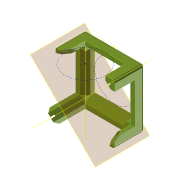
# Autodesk Inventor part: 10_Cube_1x1_v2
Saved by Autodesk Inventor 2019 (Build 230136000, 136)
## iProperties
Created: 2019-07-01
Part Number: 10_Cube_1x1_v2
Material: Generic
Document SubType Name: Modeling
Designer: diederichbenedict
Density: 1 g/cm^3
Appearance: IPHT_Grün
Author: diederichbenedict
Autodesk Inventor part; units mm, degrees
ref_plane "YZ Plane" through (0, 0, 0) normal (1, 0, 0) x (0, 1, 0)
ref_plane "XZ Plane" through (0, 0, 0) normal (0, 1, 0) x (-1, 0, 0)
sketch "Sketch1" plane through (0, 0, 0) normal (0, 0, 1) x (1, 0, 0)
  line L0 (-24.9, 24.9) -> (24.9, 24.9)
  line L1 (24.9, 24.9) -> (24.9, -24.9)
  line L2 (24.9, -24.9) -> (-24.9, -24.9)
  line L3 (-24.9, -24.9) -> (-24.9, 24.9)
  line L4 (-24.9, 24.9) -> (24.9, -24.9) construction
  line L5 (24.9, 24.9) -> (-24.9, -24.9) construction
  line L6 (16.9, 16.9) -> (-16.9, 16.9)
  line L7 (-16.9, 16.9) -> (-16.9, -16.9)
  line L8 (-16.9, -16.9) -> (16.9, -16.9)
  line L9 (16.9, -16.9) -> (16.9, 16.9)
  point P0 (0, 0)
  dimension "d0" = 49.8
  dimension "d1" = 49.8
  dimension "d2" = 8
  constraints: 20 end point, 4 parallel, 2 midpoint, 2 perpendicular, 1 horizontal, 3 other
  measures "d0" distance of L1.end L2.end
  measures "d1" distance of L0.end L1.end
  measures "d2" distance between parallel lines of L0 L6
extrude "Extrusion1" add sketch "Sketch1" along normal blind 8
sketch "Sketch2" plane through (0, 0, 8) normal (0, 0, 1) x (1, 0, 0)
  line L0 (16.9, 16.9) -> (16.9, -16.9) projected
  line L1 (16.9, -16.9) -> (-16.9, -16.9) projected
  line L2 (-16.9, -16.9) -> (-16.9, 16.9) projected
  line L3 (-16.9, 16.9) -> (16.9, 16.9) projected
  line L4 (24.9, 24.9) -> (-24.9, 24.9) projected
  line L5 (-24.9, 24.9) -> (-24.9, -24.9) projected
  line L6 (-24.9, -24.9) -> (24.9, -24.9) projected
  line L7 (24.9, -24.9) -> (24.9, 24.9) projected
  line L8 (16.9, -16.9) -> (24.9, -16.9)
  line L9 (24.9, -16.9) -> (24.9, -24.9)
  line L10 (24.9, -24.9) -> (16.9, -24.9)
  line L11 (16.9, -24.9) -> (16.9, -16.9)
  line L12 (16.9, 16.9) -> (-16.9, 16.9) projected
  line L13 (24.9, 24.9) -> (16.9, 24.9)
  line L14 (16.9, 24.9) -> (16.9, 16.9)
  line L15 (16.9, 16.9) -> (24.9, 16.9)
  line L16 (24.9, 16.9) -> (24.9, 24.9)
  line L17 (-24.9, -24.9) -> (-16.9, -24.9)
  line L18 (-16.9, -24.9) -> (-16.9, -16.9)
  line L19 (-16.9, -16.9) -> (-24.9, -16.9)
  line L20 (-24.9, -16.9) -> (-24.9, -24.9)
  line L21 (-24.9, 24.9) -> (-16.9, 24.9)
  line L22 (-16.9, 24.9) -> (-16.9, 16.9)
  line L23 (-16.9, 16.9) -> (-24.9, 16.9)
  line L24 (-24.9, 16.9) -> (-24.9, 24.9)
  point P0 (0, 0)
  constraints: 32 end point, 8 parallel, 4 horizontal, 4 perpendicular
extrude "Extrusion2" add sketch "Sketch2" along normal blind 16.9 contours L14 L4 L7 L15 | L8 L7 L6 L11 | L23 L5 L4 L22 | L18 L6 L5 L19
sketch "Sketch3" plane through (0, 0, 0) normal (0, 0, -1) x (-1, 0, 0)
  line L0 (24.9, -24.9) -> (24.9, 24.9) construction
  line L1 (24.9, 24.9) -> (-24.9, 24.9) construction
  line L2 (-24.9, -24.9) -> (24.9, -24.9) construction
  line L3 (-24.9, 24.9) -> (-24.9, -24.9) construction
  point P0 (20, 20)
  point P1 (20, -20)
  point P2 (-20, -20)
  point P3 (-20, 20)
  dimension "d_1" = 4.9
  dimension "d96" = 4.9
  dimension "d97" = 4.9
  dimension "d98" = 4.9
  dimension "d99" = 4.9
  dimension "d100" = 4.9
  dimension "d101" = 4.9
  dimension "d102" = 4.9
  measures "d_1" distance from line of L1 point (20, 20)
  measures "d96" distance from line of point (20, 20) L0
  measures "d97" distance from line of point (20, -20) L0
  measures "d98" distance from line of point (20, -20) L2
  measures "d99" distance from line of point (-20, -20) L2
  measures "d100" distance from line of point (-20, -20) L3
  measures "d101" distance from line of point (-20, 20) L3
  measures "d102" distance from line of point (-20, 20) L1
hole "Hole1" at (-20, 20, 0) at (-20, -20, 0) at (20, -20, 0) at (20, 20, 0) direction (0, 0, 1) diameter 2.8 depth 30 tip angle 118 counterbore diameter 5.5 counterbore depth 3.1
sketch "Sketch4" plane through (-24.9, 24.9, 0) normal (0, 1, 0) x (1, 0, 0)
  line L0 (0, 0) -> (49.8, 0) construction
  line L1 (0, 0) -> (0, -24.9) construction
  line L2 (8, -24.9) -> (0, -24.9) construction
  line L3 (8, -8) -> (8, -24.9) construction
  line L4 (41.8, -8) -> (8, -8) construction
  line L5 (41.8, -8) -> (41.8, -24.9) construction
  line L6 (49.8, -24.9) -> (41.8, -24.9) construction
  line L7 (49.8, 0) -> (49.8, -24.9) construction
  circle A0 centre (24.9, -24.9) radius 16.9 construction
  point P0 (24.9, 0)
  constraints: 3 tangent, 1 centre point
sketch "Sketch5" plane through (0, 0, 0) normal (0, 0, -1) x (-1, 0, 0)
  line L0 (-16.9, -16.9) -> (-16.9, 16.9) construction
  line L1 (-16.9, 16.9) -> (16.9, 16.9) construction
  line L2 (16.9, 16.9) -> (16.9, -16.9) construction
  line L3 (16.9, -16.9) -> (-16.9, -16.9) construction
  circle A0 centre (0, 0) radius 16.9 construction
  point P0 (0, 0)
  constraints: 3 tangent, 1 centre point
fillet "Fillet1" radius 2 8 edges at (24.9, 24.9, 12.45) (24.9, -24.9, 12.45) (-24.9, -24.9, 12.45) (-24.9, 24.9, 12.45) (-24.9, 0, 0) (0, -24.9, 0) (24.9, 0, 0) (0, 24.9, 0)
sketch "Sketch6" plane through (0, 0, 24.9) normal (0, 0, 1) x (1, 0, 0)
  arc A0 (-22.9, 24.9) -> (-24.9, 22.9) centre (-22.9, 22.9) ccw projected
  line L0 (-24.9, 22.9) -> (-24.9, 16.9) projected
  line L1 (-24.9, 16.9) -> (-16.9, 16.9) projected
  line L2 (-16.9, 16.9) -> (-16.9, 24.9) projected
  line L3 (-16.9, 24.9) -> (-22.9, 24.9) projected
  arc A1 (24.9, 22.9) -> (22.9, 24.9) centre (22.9, 22.9) ccw projected
  line L4 (22.9, 24.9) -> (16.9, 24.9) projected
  line L5 (16.9, 24.9) -> (16.9, 16.9) projected
  line L6 (16.9, 16.9) -> (24.9, 16.9) projected
  line L7 (24.9, 16.9) -> (24.9, 22.9) projected
  arc A2 (22.9, -24.9) -> (24.9, -22.9) centre (22.9, -22.9) ccw projected
  line L8 (24.9, -22.9) -> (24.9, -16.9) projected
  line L9 (24.9, -16.9) -> (16.9, -16.9) projected
  line L10 (16.9, -16.9) -> (16.9, -24.9) projected
  line L11 (16.9, -24.9) -> (22.9, -24.9) projected
  arc A3 (-24.9, -22.9) -> (-22.9, -24.9) centre (-22.9, -22.9) ccw projected
  line L12 (-22.9, -24.9) -> (-16.9, -24.9) projected
  line L13 (-16.9, -24.9) -> (-16.9, -16.9) projected
  line L14 (-16.9, -16.9) -> (-24.9, -16.9) projected
  line L15 (-24.9, -16.9) -> (-24.9, -22.9) projected
  line L16 (0, 38.1838) -> (54, 38.1838) construction
  line L17 (21.2838, 16.9) -> (16.9, 21.2838)
  line L18 (16.9, 24.9) -> (16.9, 16.9) projected
  line L19 (16.9, 21.2838) -> (16.9, 16.9)
  line L20 (16.9, 16.9) -> (21.2838, 16.9)
  line L21 (-16.9, 24.9) -> (-16.9, 16.9) projected
  line L22 (-16.9, 16.9) -> (-16.9, 21.2838)
  line L23 (-16.9, 21.2838) -> (-21.2838, 16.9)
  line L24 (-16.9, 21.2838) -> (-10.7004, 21.2838) construction
  line L25 (-16.9, -16.9) -> (-16.9, 16.9) projected
  line L26 (-21.2838, 16.9) -> (-16.9, 16.9)
  line L27 (-16.9, 16.9) -> (-21.2838, 16.9)
  line L28 (16.9, -16.9) -> (16.9, -24.9) projected
  line L29 (16.9, -16.9) -> (21.2838, -16.9)
  line L30 (24.9, -16.9) -> (16.9, -16.9) projected
  line L31 (21.2838, -16.9) -> (16.9, -21.2838)
  line L32 (16.9, -16.9) -> (16.9, -21.2838)
  line L33 (-16.9, -16.9) -> (-21.2838, -16.9)
  line L34 (-16.9, -16.9) -> (-16.9, -24.9) projected
  line L35 (-16.9, -16.9) -> (-16.9, -21.2838)
  line L36 (-21.2838, -16.9) -> (-16.9, -21.2838)
  dimension "d105" = 4.3838
  dimension "d106" = 4.3838
  dimension "d107" = 4.3838
  dimension "d108" = 4.3838
  dimension "d109" = 4.3838
  dimension "d110" = 4.3838
  dimension "d111" = 0
  constraints: 30 end point, 9 point on line, 3 collinear, 2 horizontal, 2 perpendicular, 1 equal length, 1 parallel, 1 vertical
  measures "d105" distance of L5.end L17.end
  measures "d106" distance of L5.end L17.start
  measures "d107" distance of L1.end L22.end
  measures "d108" distance of L23.end L1.end
  measures "d109" distance of L35.end L13.end
  measures "d110" distance of L33.end L13.end
  measures "d111" vertical distance of L35.end L31.end
extrude "Extrusion3" cut sketch "Sketch6" against normal up to surface (16.9 mm away) contours L2 L1 L23 | L6 L5 L17 | L10 L9 L31 | L14 L13 L36
sketch "Sketch7" plane through (-24.9, 16.9, 8) normal (0, -1, 0) x (1, 0, 0)
  line L0 (41.8, 0) -> (49.8, 0) construction
  line L1 (41.8, -8) -> (41.8, 0) construction
  line L2 (8, -8) -> (8, 0) construction
  line L3 (0, 0) -> (8, 0) construction
  line L4 (41.8, 33.8) -> (41.8, 0) construction
  line L5 (8, 0) -> (8, 33.8) construction
  line L6 (41.8, 0) -> (8, 0) construction
  circle A0 centre (24.9, 16.9) radius 16.9 construction
  line L7 (24.9, 54.9423) -> (-13.1423, 16.9) construction
  line L8 (-13.1423, 16.9) -> (24.9, -21.1423) construction
  line L9 (24.9, -21.1423) -> (62.9423, 16.9) construction
  line L10 (62.9423, 16.9) -> (24.9, 54.9423) construction
  line L11 (24.9, 54.9423) -> (24.9, -21.1423) construction
  line L12 (-13.1423, 16.9) -> (62.9423, 16.9) construction
  line L13 (24.9, 54.9423) -> (78.7, 54.9423) construction
  line L14 (46.1838, 0) -> (41.8, 0)
  line L15 (46.1838, 0) -> (41.8, -4.2423)
  line L16 (41.8, 0) -> (41.8, 33.8)
  line L17 (41.8, 0) -> (41.8, -4.2423)
  line L18 (46.1838, 0) -> (41.8, 0)
  line L19 (41.8, 0) -> (46.1838, 0)
  line L20 (8, 0) -> (3.6162, 0)
  line L21 (3.6162, 0) -> (8, -4.2423)
  line L22 (8, -4.2423) -> (8, 0)
  point P0 (44.386, 0)
  point P1 (43.5978, 0)
  dimension "d37" = 53.8
  dimension "d38" = 135
  dimension "d39" = 53.8
  constraints: 40 end point, 4 point on line, 3 collinear, 3 tangent, 2 horizontal, 2 midpoint, 2 parallel, 1 centre point, 1 equal length, 1 perpendicular, 1 vertical, 1 other
  measures "d37" distance of L7.start L7.end
  measures "d38" angle of L7 L13
  measures "d39" distance of L8.end L7.end
extrude "Extrusion4" cut sketch "Sketch7" along normal up to surface (33.8 mm away)
sketch "Sketch8" plane through (16.9, -24.9, 8) normal (-1, 0, 0) x (0, 0, 1)
  line L0 (-4.2423, 41.8) -> (0, 41.8) construction
  line L1 (-4.2423, 8) -> (0, 8) construction
  line L2 (0, 8) -> (0, 3.6162) construction
  line L3 (-4.2423, 8) -> (0, 3.6162)
  line L4 (0, 3.6162) -> (0, 8)
  line L5 (0, 8) -> (-4.2423, 8)
  line L6 (-4.2423, 41.8) -> (0, 46.0423)
  line L7 (-4.2423, 41.8) -> (1.7572, 41.8) construction
  line L8 (0, 8) -> (0, 41.8)
  line L9 (0, 46.0423) -> (0, 41.8)
  line L10 (0, 41.8) -> (-4.2423, 41.8)
  line L11 (-6, 2) -> (-6, 47.8)
  point P0 (-2.4341, 8)
  point P1 (0, 5.414)
  dimension "d112" = 45
  constraints: 24 end point, 2 vertical, 1 collinear, 1 equal length, 1 horizontal, 1 perpendicular
  measures "d112" angle of L7 L6
ref_plane "Work Plane1" through (-20.32, -18.034, 19.8181) normal (-1, 0, 0) x (0, 0, 1)
extrude "Extrusion5" cut sketch "Sketch8" along normal up to surface (33.8 mm away)
ref_plane "Work Plane2" through (0.3941, -0.3941, 8) normal (0.7071068, 0.7071068, 0) x (-0.7071068, 0.7071068, 0)
ref_plane "Work Plane3" through (-0.3941, -0.3941, 24.9) normal (0.7071068, -0.7071068, 0) x (-0.7071068, -0.7071068, 0)
sketch "Sketch16" plane through (0.3941, -0.3941, 8) normal (0.7071068, 0.7071068, 0) x (-0.7071068, 0.7071068, 0)
  line L0 (1.9716, -6) -> (1.9716, 16.9) projected
  line L1 (34.3571, -6) -> (1.9716, -6) projected
  line L2 (34.3571, 16.9) -> (34.3571, -6) projected
  line L3 (30.1144, 16.9) -> (34.3571, 16.9) projected
  line L4 (30.1144, 0) -> (30.1144, 16.9) projected
  line L5 (6.2142, 0) -> (30.1144, 0) projected
  line L6 (6.2142, 0) -> (6.2142, 16.9) projected
  line L7 (1.9716, 16.9) -> (6.2142, 16.9) projected
  line L8 (27.5574, 16.9) -> (30.2416, 16.9) projected
  line L9 (27.5574, 16.9) -> (32.5574, 16.9)
  line L10 (27.5574, 16.9) -> (27.5574, 6.9)
  line L11 (27.5574, 16.9) -> (37.5574, 16.9) construction
  line L12 (27.5574, 6.9) -> (32.5574, 16.9)
  point P0 (0.5574, -8)
  dimension "d115" = 5
  dimension "d116" = 10
  dimension "d117" = 90
  constraints: 8 end point, 1 horizontal, 1 perpendicular, 1 point on line, 1 vertical
  measures "d115" distance of L8.start L9.end
  measures "d116" distance of L8.start L10.end
  measures "d117" angle of L10 L11
extrude "Extrusion6" cut sketch "Sketch16" along normal through all both and the other way through all contours L12 L4 L3 | L12 L10 L8 L4
mirror "Mirror1" about plane through (-0.3941, -0.3941, 24.9) normal (0.7071068, -0.7071068, 0) of "Extrusion6"
sketch "Sketch17" plane through (0, 0, 24.9) normal (0, 0, 1) x (1, 0, 0)
  line L0 (-19.486, -18.6978) -> (-21.2838, -16.9) projected
  line L1 (-21.2838, -16.9) -> (-24.9, -16.9) projected
  line L2 (-24.9, -16.9) -> (-24.9, -22.9) projected
  arc A0 (-24.9, -22.9) -> (-22.9, -24.9) centre (-22.9, -22.9) ccw projected
  line L3 (-22.9, -24.9) -> (-16.9, -24.9) projected
  line L4 (-16.9, -24.9) -> (-16.9, -21.2838) projected
  line L5 (-16.9, -21.2838) -> (-18.6978, -19.486) projected
  arc A1 (-19.486, -18.6978) -> (-18.6978, -19.486) centre (-20, -20) ccw projected
  line L6 (19.486, 18.6978) -> (21.2838, 16.9) projected
  line L7 (21.2838, 16.9) -> (24.9, 16.9) projected
  line L8 (24.9, 16.9) -> (24.9, 22.9) projected
  arc A2 (24.9, 22.9) -> (22.9, 24.9) centre (22.9, 22.9) ccw projected
  line L9 (22.9, 24.9) -> (16.9, 24.9) projected
  line L10 (16.9, 24.9) -> (16.9, 21.2838) projected
  line L11 (16.9, 21.2838) -> (18.6978, 19.486) projected
  arc A3 (19.486, 18.6978) -> (18.6978, 19.486) centre (20, 20) ccw projected
  line L12 (-24.9, 16.9) -> (-24.9, 20.3548) projected
  line L13 (-21.2838, 16.9) -> (-24.9, 16.9) projected
  line L14 (-19.486, 18.6978) -> (-21.2838, 16.9) projected
  arc A4 (-18.6978, 19.486) -> (-19.486, 18.6978) centre (-20, 20) ccw projected
  line L15 (-16.9, 21.2838) -> (-18.6978, 19.486) projected
  line L16 (-16.9, 24.9) -> (-16.9, 21.2838) projected
  line L17 (-20.3548, 24.9) -> (-16.9, 24.9) projected
  line L18 (-24.9, 20.3548) -> (-20.3548, 24.9) projected
  line L19 (20.3548, -24.9) -> (16.9, -24.9) projected
  line L20 (24.9, -20.3548) -> (20.3548, -24.9) projected
  line L21 (24.9, -16.9) -> (24.9, -20.3548) projected
  line L22 (21.2838, -16.9) -> (24.9, -16.9) projected
  line L23 (19.486, -18.6978) -> (21.2838, -16.9) projected
  arc A5 (18.6978, -19.486) -> (19.486, -18.6978) centre (20, -20) ccw projected
  line L24 (16.9, -21.2838) -> (18.6978, -19.486) projected
  line L25 (16.9, -24.9) -> (16.9, -21.2838) projected
  line L26 (-21.2838, 16.9) -> (-16.9, 16.9) projected
  line L27 (-16.9, 16.9) -> (-16.9, 21.1423) projected
  line L28 (16.9, -16.9) -> (16.9, -21.2838) projected
  line L29 (21.2838, -16.9) -> (16.9, -16.9) projected
  line L30 (-24.9, -20.3548) -> (-20.3548, -24.9) construction
  line L31 (-24.7939, -20.2488) -> (-20.2488, -24.7939) construction
  line L32 (-24.9, -22.9) -> (-24.9, 22.9) projected
  line L33 (-24.9, -20.1427) -> (-20.1427, -24.9)
  line L34 (22.9, -24.9) -> (-22.9, -24.9) projected
  point P0 (0, 0)
  dimension "d120" = 0.15
  constraints: 6 end point, 2 point on line, 1 parallel, 3 other
  measures "d120" distance between parallel lines of L30 L31
extrude "Extrusion7" add sketch "Sketch17" along normal blind 10 contours A1 L5 L4 L3 L33 L2 L1 L0
ref_plane "Work Plane4" through (-16.9, -16.9, 8) normal (-0.7071068, 0.7071068, 0) x (0, 0, 1)
sketch "Sketch18" plane through (-0.3941, -0.3941, 24.9) normal (0.7071068, -0.7071068, 0) x (-0.7071068, -0.7071068, 0)
  line L0 (28.9997, -4.8859) -> (31.4426, 0)
  line L1 (33.2423, 0) -> (31.4426, 0)
  line L2 (26.4426, -10) -> (28.9997, -4.8859)
  line L3 (31.2926, -10) -> (28.9997, -10) projected
  line L4 (26.4426, -10) -> (31.2926, -10)
  line L5 (31.2926, -10) -> (31.2926, -0.3)
  line L6 (31.2926, 0) -> (31.2926, -10) projected
  point P0 (-0.5574, 24.9)
  constraints: 10 end point, 2 horizontal, 2 point on line, 6 other
extrude "Extrusion8" cut sketch "Sketch18" along normal through all both and the other way through all
mirror "Mirror2" about plane through (0.3941, -0.3941, 8) normal (0.7071068, 0.7071068, 0) of "Extrusion8", "Extrusion7"
equation "\"d96\" = d_1"
equation "\"d97\" = d_1"
equation "\"d98\" = d_1"
equation "\"d99\" = d_1"
equation "\"d100\" = d_1"
equation "\"d101\" = d_1"
equation "\"d102\" = d_1"
body "Solid1"
